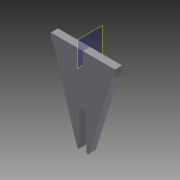
# Autodesk Inventor part: brace03
Saved by Autodesk Inventor 2013 (Build 170138000, 138)
## iProperties
Created: 2013-09-17
Part Number: brace03
Material: Generic
Document SubType Name: Modeling
Designer: Nano
Density: 1 g/cm^3
Author: Nano
Autodesk Inventor part; units mm, degrees
ref_plane "YZ Plane" through (0, 0, 0) normal (1, 0, 0) x (0, 1, 0)
ref_plane "XZ Plane" through (0, 0, 0) normal (0, 1, 0) x (-1, 0, 0)
ref_plane "XY Plane" through (0, 0, 0) normal (0, 0, 1) x (1, 0, 0)
sketch "Sketch1" plane through (0, 0, 0) normal (0, 0, 1) x (1, 0, 0)
  line L0 (-3.175, -49.7295) -> (-3.175, -11.6295)
  line L1 (-3.175, -11.6295) -> (3.175, -11.6295)
  line L2 (3.175, -11.6295) -> (3.175, -49.7295)
  line L3 (3.175, -49.7295) -> (28.575, 33.5996)
  line L4 (28.575, 33.5996) -> (-28.575, 33.5996)
  line L5 (-28.575, 33.5996) -> (-3.175, -49.7295)
  line L6 (0, -0.0188) -> (0, -58.4605) construction
  point P0 (0, 0)
  dimension "d3" = 6.35
  dimension "d4" = 38.1
  dimension "d5" = 38.1
  dimension "d6" = 90
  dimension "d7" = 90
  dimension "d12" = 45.2291
  dimension "d13" = 57.15
  dimension "d14" = 83.3291
  dimension "d15" = 17.5367
  dimension "d16" = 3.175
  dimension "d17" = 33.6184
  dimension "d18" = 92.0601
  constraints: 14 end point, 1 parallel, 1 perpendicular, 1 other
  measures "d3" distance of L0.end L1.end
  measures "d4" distance of L0.start L0.end
  measures "d5" distance of L1.end L2.end
  measures "d6" angle of L0 L1
  measures "d7" angle of L1 L2
  measures "d12" distance between parallel lines of L4 L1
  measures "d13" distance of L3.end L4.end
  measures "d14" vertical distance of L2.end L3.end
  measures "d15" distance from line of point (0, 0) L3
  measures "d16" distance from line of point (0, 0) L2
  measures "d17" distance from line of L6.start L4
  measures "d18" distance from line of L6.end L4
extrude "Extrusion1" add sketch "Sketch1" along normal blind 6.35
sketch "Sketch2" plane through (28.575, 33.5996, 6.35) normal (0.9565492, -0.2915711, 0) x (0, 0, -1)
  line L0 (6.35, 0) -> (0, 0) projected
  line L1 (6.35, -6.35) -> (0, -6.35)
  line L2 (0, -6.35) -> (0, 0)
  line L3 (0, 0) -> (6.35, 0)
  line L4 (6.35, 0) -> (6.35, -6.35)
  point P0 (6.35, -40.4713)
  dimension "d19" = 6.35
  dimension "d21" = 6.35
  constraints: 8 end point, 2 parallel, 1 horizontal, 1 perpendicular
  measures "d19" distance of L3.end L1.start
  measures "d21" distance of L1.start L1.end
revolve "Revolution1" add sketch "Sketch2" angle 17 about axis through (28.575, 33.5996, 0) along (0, 0, 1)
fillet "Fillet1" radius 3.175 1 edges at (26.7235, 27.5255, 3.175)
ref_plane "Work Plane1" through (0, 33.5996, 0) normal (-1, 0, 0) x (0, -1, 0)
mirror "Mirror1" about plane through (0, 33.5996, 0) normal (-1, 0, 0) of "Revolution1"
fillet "Fillet2" radius 3.175 1 edges at (-26.7235, 27.5255, 3.175)
fillet "Fillet3" radius 1.016 2 edges at (-3.175, -49.7295, 3.175) (3.175, -49.7295, 3.175)
body "Solid1"
